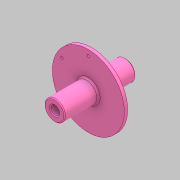
# Autodesk Inventor part: EncoderDisk
Saved by Autodesk Inventor 2018 (Build 220112000, 112)
## iProperties
Created: 2019-06-28
Part Number: EncoderDisk
Material: Generic
Document SubType Name: Modeling
Designer: mkivekas
Density: 1 g/cm^3
Appearance: Pink
Mass: 3.21765 g
Surface Area: 34.3373 cm^2
Volume: 3.21765 cm^3
Author: mkivekas
Autodesk Inventor part; units mm, degrees
ref_plane "XZ Plane" through (0, 0, 0) normal (0, 1, 0) x (-1, 0, 0)
sketch "Sketch1" plane through (0, 0, 0) normal (0, 1, 0) x (-1, 0, 0)
  circle A0 centre (0, 0) radius 21.25
  circle A1 centre (0, 0) radius 18
  point P0 (0, 18)
  point P1 (15.4613, 9.2168)
  dimension "d0" = 42.5
  dimension "d3" = 3.25
  dimension "d4" = 59.2
  constraints: 3 coincident, 2 centre point, 2 point on circle
  measures "d0" diameter of A0
  measures "d3" radial gap between concentric circles of A0 A1
extrude "Extrusion1" add sketch "Sketch1" along normal blind 2 contours A0 | A1
hole "Hole1" at (0, 0, 18) at (-15.4613, 0, 9.2168) direction (0, 1, 0) diameter 1.5 depth 8 tip angle 118
sketch "Sketch2" plane through (0, 0, 0) normal (0, -1, 0) x (1, 0, 0)
  circle A0 centre (0, 0) radius 6
  dimension "d19" = 12
  constraints: 1 centre point, 1 coincident
  measures "d19" diameter of A0
extrude "Extrusion2" add sketch "Sketch2" along normal blind 20 and the other way blind 22
chamfer "Chamfer2" distance 0.5 angle 45 2 edges at (-6, 22, 0) (-6, -20, 0)
fillet "Fillet1" radius 1 2 edges at (-6, 0, 0) (-6, 2, 0)
sketch "Sketch3" plane through (0, -20, 0) normal (0, -1, 0) x (1, 0, 0)
  point P0 (0, 0)
  point P1 (0, 0)
  constraints: 1 coincident
hole "Hole3" at (0, -20, 0) direction (0, 1, 0) diameter 5.1 end through all
chamfer "Chamfer3" distance 0.5 angle 45 2 edges at (0, -20, 2.55) (0, 22, 2.55)
ref_plane "Work Plane1" through (-6, 0, 0) normal (1, 0, 0) x (0, 1, 0)
sketch "Sketch4" plane through (-6, 0, 0) normal (1, 0, 0) x (0, 1, 0)
  line L0 (22, 5.5) -> (22, -5.5) projected
  line L1 (-20, -5.5) -> (-20, 5.5) projected
  point P0 (0, 0)
  point P1 (17, 0)
  point P2 (-15, 0)
  dimension "d41" = 5
  dimension "d42" = 5
  measures "d41" distance from line of L0 point (17, 0)
  measures "d42" distance from line of L1 point (-15, 0)
ref_plane "Work Plane2" through (0, 0, -6) normal (0, 0, 1) x (1, 0, 0)
sketch "Sketch6" plane through (0, 0, -6) normal (0, 0, 1) x (1, 0, 0)
  line L0 (5.5, -20) -> (-5.5, -20) projected
  line L1 (-5.5, 22) -> (5.5, 22) projected
  point P0 (0, 0)
  point P1 (0, -15)
  point P2 (0, 17)
  dimension "d43" = 5
  dimension "d44" = 5
  measures "d43" distance from line of L0 point (0, -15)
  measures "d44" distance from line of L1 point (0, 17)
hole "Hole4" at (-6, -15, 0) at (-6, 17, 0) direction (1, 0, 0) diameter 2.459 depth 5.8 tip angle 118 thread size "M3x0.5" class "6H" standard "ISO Metric profile"
hole "Hole5" at (0, -15, -6) at (0, 17, -6) direction (0, 0, 1) diameter 2.459 depth 5.8 tip angle 118 thread size "M3x0.5" class "6H" standard "ISO Metric profile"
body "Solid1"
